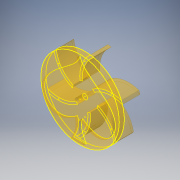
# Autodesk Inventor part: s_fan
Saved by Autodesk Inventor 2016 (Build 200138000, 138)
## iProperties
Created: 2016-08-31
Part Number: s_fan
Material: 一般
Document SubType Name: Modeling
Designer: KOTA-NPC2
Density: 1 g/cm^3
Appearance: ポリカーボネート - クリア
Author: KOTA-NPC2
Autodesk Inventor part; units mm, degrees
ref_plane "YZ Plane" through (0, 0, 0) normal (1, 0, 0) x (0, 1, 0)
ref_plane "XZ Plane" through (0, 0, 0) normal (0, 1, 0) x (-1, 0, 0)
ref_plane "XY Plane" through (0, 0, 0) normal (0, 0, 1) x (1, 0, 0)
ref_plane "作業平面4" through (0, 0, 0.5) normal (0, 0, 1) x (1, 0, 0)
sketch "スペード" plane through (0, 0, 0.5) normal (0, 0, 1) x (1, 0, 0)
  spline S0 degree 4 poles (0, 22) (-0.5767, 17.9676) (-14.0465, 11.4325) (-18.1981, 5.212) (-9.6108, -5.2964) (-1, 1) knots 0 0 0 0 0 0.493807 1 1 1 1 1
  spline S1 degree 4 poles (0, 22) (0.5767, 17.9676) (14.0465, 11.4325) (18.1981, 5.212) (9.6108, -5.2964) (1, 1) knots 0 0 0 0 0 0.493807 1 1 1 1 1
  spline S2 degree 2 poles (1, 1) (-0.3805, -2.1136) (2.5, -7) knots 0 0 0 1 1 1
  spline S3 degree 2 poles (-1, 1) (0.3805, -2.1136) (-2.5, -7) knots 0 0 0 1 1 1
  line L0 (-2.5, -7) -> (2.5, -7)
  circle A0 centre (0, 7) radius 15.5
  circle A1 centre (0, 7) radius 1
  point P0 (0, 0)
  point P1 (-5, 16)
  point P2 (-12, 10)
  point P3 (-14, 5)
  point P4 (5, 16)
  point P5 (12, 10)
  point P6 (14, 5)
  point P7 (-12, 0)
  point P8 (12, 0)
  point P9 (0.6, -2)
  point P10 (-0.6, -2)
  dimension "d180" = 5
  dimension "d181" = 5
  dimension "d182" = 12
  dimension "d183" = 12
  dimension "d184" = 14
  dimension "d185" = 14
  dimension "d186" = 12
  dimension "d187" = 12
  dimension "d188" = 21
  dimension "d189" = 21
  dimension "d190" = 6
  dimension "d191" = 0
  dimension "d192" = 6
  dimension "d193" = 1
  dimension "d194" = 1
  dimension "d195" = 6
  dimension "d196" = 6
  dimension "d197" = 5
  dimension "d198" = 5
  dimension "d199" = 5
  dimension "d200" = 5
  dimension "d202" = 22
  dimension "d203" = 0.6
  dimension "d204" = 2.5
  dimension "d206" = 0.6
  dimension "d207" = 2.5
  dimension "d208" = 8
  dimension "d209" = 3
  dimension "d210" = 3
  dimension "d251" = 31
  dimension "d252" = 15
  dimension "d253" = 0
  dimension "d258" = 2
  constraints: 2 centre point, 2 end point, 1 coincident, 1 horizontal, 18 other
  measures "d180" horizontal distance of point (0, 0) point (-5, 16)
  measures "d181" horizontal distance of point (0, 0) point (5, 16)
  measures "d182" horizontal distance of point (0, 0) point (-12, 10)
  measures "d183" horizontal distance of point (0, 0) point (12, 10)
  measures "d184" horizontal distance of point (0, 0) point (-14, 5)
  measures "d185" horizontal distance of point (0, 0) point (14, 5)
  measures "d186" distance of point (0, 0) point (-12, 0)
  measures "d187" distance of point (0, 0) point (12, 0)
  measures "d188" vertical distance of point (-1, 1) point (0, 22)
  measures "d189" vertical distance of point (1, 1) point (0, 22)
  measures "d190" vertical distance of point (-5, 16) point (0, 22)
  measures "d191" horizontal distance of point (0, 0) point (0, 22)
  measures "d192" vertical distance of point (0, 22) point (5, 16)
  measures "d193" horizontal distance of point (0, 0) point (-1, 1)
  measures "d194" horizontal distance of point (0, 0) point (1, 1)
  measures "d195" vertical distance of point (12, 10) point (5, 16)
  measures "d196" vertical distance of point (-5, 16) point (-12, 10)
  measures "d197" vertical distance of point (-14, 5) point (-12, 10)
  measures "d198" vertical distance of point (14, 5) point (12, 10)
  measures "d199" vertical distance of point (-12, 0) point (-14, 5)
  measures "d200" vertical distance of point (12, 0) point (14, 5)
  measures "d202" distance of point (0, 0) point (0, 22)
  measures "d203" horizontal distance of point (0, 0) point (0.6, -2)
  measures "d204" horizontal distance of L0.end point (0, 0)
  measures "d206" horizontal distance of point (0, 0) point (-0.6, -2)
  measures "d207" horizontal distance of point (0, 0) L0.start
  measures "d208" distance from line of L0 point (-1, 1)
  measures "d209" vertical distance of point (1, 1) point (0.6, -2)
  measures "d210" vertical distance of point (-0.6, -2) point (-1, 1)
  measures "d251" diameter of A0
  measures "d252" distance of A0.centre point (0, 22)
  measures "d253" horizontal distance of point (0, 22) A0.centre
  measures "d258" diameter of A1
extrude "押し出し14" add sketch "スペード" against normal blind 2 contours S1 S2 L0 S3 S0 | A0
extrude "押し出し15" add sketch "スペード" along normal blind 1 contours S1 S2 L0 S3 S0
sketch "スケッチ19" plane through (0, 7, -1.5) normal (0, 0, -1) x (-1, 0, 0)
  circle A0 centre (0, 0) radius 15.5 construction
  circle A1 centre (0, 12) radius 12 construction
  line L0 (0, 0) -> (0, 29.6691) construction
  circle A2 centre (0, 0) radius 5 construction
  arc A3 (4.7598, 1.5313) -> (11.4018, 10.5) centre (0, 12) ccw
  arc A4 (4.9717, 0.5313) -> (12.2474, 9.5) centre (0, 12) ccw
  arc A5 (4.9717, 0.5313) -> (4.7598, 1.5313) centre (0, 0) ccw
  arc A6 (12.2474, 9.5) -> (11.4018, 10.5) centre (0, 0) ccw
  arc A7 (-2.1035, 15.3566) -> (-3.3924, 15.1242) centre (0, 0) ccw
  arc A8 (1.0538, 4.8877) -> (-3.3924, 15.1242) centre (-10.3923, 6) ccw
  arc A9 (2.0258, 4.5712) -> (-2.1035, 15.3566) centre (-10.3923, 6) ccw
  arc A10 (2.0258, 4.5712) -> (1.0538, 4.8877) centre (0, 0) ccw
  arc A11 (-14.351, 5.8566) -> (-14.7941, 4.6242) centre (0, 0) ccw
  arc A12 (-3.706, 3.3564) -> (-14.7941, 4.6242) centre (-10.3923, -6) ccw
  arc A13 (-2.9459, 4.04) -> (-14.351, 5.8566) centre (-10.3923, -6) ccw
  arc A14 (-2.9459, 4.04) -> (-3.706, 3.3564) centre (0, 0) ccw
  arc A15 (-12.2474, -9.5) -> (-11.4018, -10.5) centre (0, 0) ccw
  arc A16 (-4.7598, -1.5312) -> (-11.4018, -10.5) centre (0, -12) ccw
  arc A17 (-4.9717, -0.5312) -> (-12.2474, -9.5) centre (0, -12) ccw
  arc A18 (-4.9717, -0.5312) -> (-4.7598, -1.5312) centre (0, 0) ccw
  arc A19 (2.1035, -15.3566) -> (3.3924, -15.1242) centre (0, 0) ccw
  arc A20 (-1.0538, -4.8877) -> (3.3924, -15.1242) centre (10.3923, -6) ccw
  arc A21 (-2.0258, -4.5712) -> (2.1035, -15.3566) centre (10.3923, -6) ccw
  arc A22 (-2.0258, -4.5712) -> (-1.0538, -4.8877) centre (0, 0) ccw
  arc A23 (14.351, -5.8566) -> (14.7941, -4.6242) centre (0, 0) ccw
  arc A24 (3.706, -3.3564) -> (14.7941, -4.6242) centre (10.3923, 6) ccw
  arc A25 (2.9459, -4.04) -> (14.351, -5.8566) centre (10.3923, 6) ccw
  arc A26 (2.9459, -4.04) -> (3.706, -3.3564) centre (0, 0) ccw
  point P0 (0, -7)
  dimension "d270" = 24
  dimension "d271" = 0
  dimension "d272" = 10
  dimension "d273" = 11.5
  dimension "d274" = 12.5
  dimension "d283" = 360
  constraints: 52 point on circle, 25 centre point, 10 coincident, 2 concentric, 2 end point, 2 vertical, 1 vertical alignment, 74 other
  measures "d271" horizontal distance of L0.start point (0, 12)
  measures "d272" diameter of A2
  measures "d273" radius of A3
  measures "d274" radius of A4
extrude "押し出し17" add sketch "スケッチ19" along normal blind 7
sketch "羽2" plane through (0, 7, 0.5) normal (0, 0, 1) x (1, 0, 0)
  line L0 (2.5, -14) -> (-2.5, -14) projected
  circle A0 centre (0, 0) radius 15.5 projected
  point P0 (0, -7)
  constraints: 4 other
